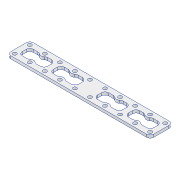
# Autodesk Inventor part: Gusset
Saved by Autodesk Inventor 2020 (Build 240168000, 168)
## iProperties
Created: 2019-12-29
Part Number: Gusset
Material: Aluminum 6061
Document SubType Name: Modeling
Designer: pchild
Density: 2.7 g/cm^3
Appearance: Aluminum - Flat
Mass: 7.58757 g
Surface Area: 37.3667 cm^2
Volume: 2.81021 cm^3
Author: pchild
Autodesk Inventor part; units mm, degrees
ref_plane "YZ Plane" through (0, 0, 0) normal (1, 0, 0) x (0, 1, 0)
ref_plane "XZ Plane" through (0, 0, 0) normal (0, 1, 0) x (-1, 0, 0)
sketch "Sketch1" plane through (0, 0, 0) normal (0, 1, 0) x (-1, 0, 0)
  circle A0 centre (0, 3.1864) radius 1.5875
  arc A1 (-3.175, 3.1864) -> (0, 6.3614) centre (0, 3.1864) ccw construction
  line L0 (57.15, 9.5364) -> (-3.175, 9.5364) construction
  line L1 (-3.175, 9.5364) -> (-3.175, -15.8636) construction
  line L2 (4.7625, 1.5989) -> (8.4999, 1.5989)
  line L3 (57.15, 6.3614) -> (0, 6.3614)
  line L4 (0, 6.3614) -> (0, 1.5989) construction
  arc A2 (15.4496, 1.5989) -> (9.9504, 1.5989) centre (12.7, 3.1864) ccw construction
  circle A3 centre (12.7, 3.1864) radius 1.5875
  circle A4 centre (25.4, 3.1864) radius 1.5875
  arc A5 (28.1496, 1.5989) -> (22.6504, 1.5989) centre (25.4, 3.1864) ccw construction
  circle A6 centre (38.1, 3.1864) radius 1.5875
  arc A7 (40.8496, 1.5989) -> (35.3504, 1.5989) centre (38.1, 3.1864) ccw construction
  circle A8 centre (0, -9.5136) radius 1.5875
  arc A9 (0, -12.6886) -> (-3.175, -9.5136) centre (0, -9.5136) ccw construction
  line L5 (1.5875, 3.1864) -> (-3.175, 3.1864) construction
  line L6 (-3.175, 3.1864) -> (-3.175, -9.5136)
  line L7 (-3.175, -9.5136) -> (1.5875, -9.5136) construction
  line L8 (1.5875, -4.7511) -> (1.5875, -1.5761)
  line L9 (57.15, 9.5364) -> (57.15, 8.3839) construction
  circle A10 centre (12.7, -9.5136) radius 1.5875
  circle A11 centre (25.4, -9.5136) radius 1.5875
  arc A12 (9.9504, -7.9261) -> (15.4496, -7.9261) centre (12.7, -9.5136) ccw construction
  line L10 (4.7625, -7.9261) -> (8.4999, -7.9261)
  line L11 (0, -12.6886) -> (0, -7.9261) construction
  arc A13 (4.7625, 1.5989) -> (1.5875, -1.5761) centre (4.7625, -1.5761) ccw
  arc A14 (1.5875, -4.7511) -> (4.7625, -7.9261) centre (4.7625, -4.7511) ccw
  arc A15 (10.5999, 0.8052) -> (14.8001, 0.8052) centre (12.7, 3.1864) ccw
  arc A16 (14.8001, -7.1323) -> (10.5999, -7.1323) centre (12.7, -9.5136) ccw
  line L12 (16.9001, 1.5989) -> (19.8438, 1.5989)
  line L13 (16.9001, -7.9261) -> (19.8438, -7.9261)
  arc A17 (10.5999, 0.8052) -> (8.4999, 1.5989) centre (8.4999, -1.5761) ccw
  arc A18 (16.9001, 1.5989) -> (14.8001, 0.8052) centre (16.9001, -1.5761) ccw
  arc A19 (8.4999, -7.9261) -> (10.5999, -7.1323) centre (8.4999, -4.7511) ccw
  arc A20 (14.8001, -7.1323) -> (16.9001, -7.9261) centre (16.9001, -4.7511) ccw
  arc A21 (-3.175, -9.5136) -> (0, -12.6886) centre (0, -9.5136) ccw
  arc A22 (0, 6.3614) -> (-3.175, 3.1864) centre (0, 3.1864) ccw
  line L14 (54.7687, 9.5364) -> (54.7688, -7.9261) construction
  line L15 (27.7812, 3.1864) -> (23.0188, 3.1864) construction
  line L16 (23.0188, -1.5761) -> (23.0188, -4.7511)
  arc A23 (23.0188, -1.5761) -> (19.8438, 1.5989) centre (19.8438, -1.5761) ccw
  arc A24 (19.8438, -7.9261) -> (23.0188, -4.7511) centre (19.8438, -4.7511) ccw
  line L17 (57.15, -12.6886) -> (0, -12.6886)
  line L18 (57.15, 6.3614) -> (57.15, -12.6886)
  line L19 (57.15, 6.8462) -> (57.15, 4.0771) construction
  line L20 (57.15, 4.0771) -> (57.15, -12.6886)
  line L21 (57.15, -0.4038) -> (57.15, -12.6886) construction
  circle A25 centre (38.1, -9.5136) radius 1.5875
  circle A26 centre (50.8, 3.1864) radius 1.5875
  circle A27 centre (50.8, -9.5136) radius 1.5875
  line L22 (25.4, 3.1864) -> (25.4, -9.5136) construction
  line L23 (46.0375, 1.5989) -> (42.3001, 1.5989)
  line L24 (49.2125, -4.7511) -> (49.2125, -1.5761)
  line L25 (46.0375, -7.9261) -> (42.3001, -7.9261)
  arc A28 (49.2125, -1.5761) -> (46.0375, 1.5989) centre (46.0375, -1.5761) ccw
  arc A29 (46.0375, -7.9261) -> (49.2125, -4.7511) centre (46.0375, -4.7511) ccw
  arc A30 (35.9999, 0.8052) -> (40.2001, 0.8052) centre (38.1, 3.1864) ccw
  arc A31 (40.2001, -7.1323) -> (35.9999, -7.1323) centre (38.1, -9.5136) ccw
  line L26 (33.8999, 1.5989) -> (30.9562, 1.5989)
  line L27 (33.8999, -7.9261) -> (30.9562, -7.9261)
  arc A32 (42.3001, 1.5989) -> (40.2001, 0.8052) centre (42.3001, -1.5761) ccw
  arc A33 (35.9999, 0.8052) -> (33.8999, 1.5989) centre (33.8999, -1.5761) ccw
  arc A34 (40.2001, -7.1323) -> (42.3001, -7.9261) centre (42.3001, -4.7511) ccw
  arc A35 (33.8999, -7.9261) -> (35.9999, -7.1323) centre (33.8999, -4.7511) ccw
  line L28 (27.7812, -1.5761) -> (27.7812, -4.7511)
  arc A36 (30.9562, 1.5989) -> (27.7812, -1.5761) centre (30.9562, -1.5761) ccw
  arc A37 (27.7812, -4.7511) -> (30.9562, -7.9261) centre (30.9562, -4.7511) ccw
  point P0 (12.7, -12.6886)
  point P1 (57.15, -9.5136)
  dimension "d23" = 3.175
  dimension "d24" = 6.35
  dimension "d26" = 25.4
  dimension "d27" = 6.35
  dimension "d28" = 12.7
  dimension "d29" = 12.7
  dimension "d30" = 12.7
  dimension "d32" = 12.7
  dimension "d34" = 3.175
  dimension "d35" = 3.175
  dimension "d37" = 2.3813
  dimension "d54" = 2.3813
  dimension "d55" = 90
  dimension "d58" = 12.7
  dimension "d59" = 60.325
  constraints: 60 point on circle, 56 end point, 36 centre point, 30 point on line, 26 symmetric about line, 22 equal radius, 16 tangent, 10 parallel, 9 horizontal alignment, 8 coincident, 7 horizontal, 7 vertical alignment, 3 perpendicular, 2 vertical, 1 midpoint, 28 other
  measures "d24" diameter of A1
  measures "d26" distance of L1.end L0.end
  measures "d27" distance from line of point (0, 3.186) L0
  measures "d28" distance of A2.centre point (0, 3.186)
  measures "d29" distance of A4.centre A2.centre
  measures "d30" distance of A6.centre A4.centre
  measures "d32" distance of A1.centre point (0, -9.514)
  measures "d34" radius of A13
  measures "d35" radius of A17
  measures "d37" distance between parallel lines of L9 L14
  measures "d54" distance from line of A4.centre L16
  measures "d55" angle of L3 L18
  measures "d58" distance of A26.centre A6.centre
  measures "d59" distance from line of L17.start L1
extrude "Extrusion1" add sketch "Sketch1" along normal blind 2.286
ref_plane "Work Plane1" through (-57.15, 1.143, 6.3614) normal (-1, 0, 0) x (0, 0, 1)
mirror "Mirror1" about plane through (-57.15, 1.143, 6.3614) normal (-1, 0, 0) of "Extrusion1"
chamfer "Chamfer1" [suppressed]
fillet "Fillet3" [suppressed]
chamfer "Chamfer3" [suppressed]
fillet "Fillet4" [suppressed]
equation "\"d29\" = d28"
equation "\"d30\" = d29"
equation "\"ANGLE\" = 180deg"
equation "\"CHAMFER\" = 11.51669"
equation "\"INNER\" = 2.286"
body "Solid1"
